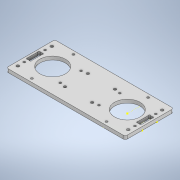
# Autodesk Inventor part: Trunk_waisit_frame_
Saved by Autodesk Inventor 2020.4 (Build 244396000, 396)
## iProperties
Created: 2021-12-30
Part Number: Trunk_waisit_frame_
Material: アルミニウム 2014-T4
Document SubType Name: Modeling
Designer: Masato Kubotera
Density: 2.8 g/cm^3
Appearance: 滑らか - 淡い灰色
Mass: 70.4243 g
Surface Area: 159.281 cm^2
Volume: 25.1515 cm^3
Author: Masato Kubotera
Autodesk Inventor part; units mm, degrees
ref_plane "YZ Plane" through (0, 0, 0) normal (1, 0, 0) x (0, 1, 0)
ref_plane "XZ Plane" through (0, 0, 0) normal (0, 1, 0) x (-1, 0, 0)
ref_plane "XY Plane" through (0, 0, 0) normal (0, 0, 1) x (1, 0, 0)
derived "Outer_support_stand.ipt"
sketch "スケッチ1" plane through (0, 0, 0) normal (0, 0, 1) x (1, 0, 0)
  circle A0 centre (0, 0) radius 18.5 construction
  circle A1 centre (0, 0) radius 20.5 construction
  circle A2 centre (0, 0) radius 20.51 construction
  line L0 (0, 0) -> (0, 24.5) construction
  circle A3 centre (0, 24.5) radius 1.55 construction
  circle A4 centre (0, 24.5) radius 3 construction
  arc A5 (0, 28.5) -> (-3.7147, 25.9835) centre (0, 24.5) ccw construction
  arc A6 (-5.1639, 24.7674) -> (-18.8673, 16.8557) centre (0, 0) ccw construction
  arc A7 (-5.1639, 24.7674) -> (-3.7147, 25.9835) centre (-5.5721, 26.7253) ccw construction
  arc A8 (3.7147, 25.9835) -> (5.1639, 24.7674) centre (5.5721, 26.7253) ccw construction
  arc A9 (3.7147, 25.9835) -> (0, 28.5) centre (0, 24.5) ccw construction
  circle A10 centre (0, 24.5) radius 3.05 construction
  arc A11 (-24.0311, 7.9117) -> (-24.0311, -7.9117) centre (0, 0) ccw construction
  arc A12 (-24.0311, 7.9117) -> (-24.3598, 9.7747) centre (-25.9308, 8.5371) ccw construction
  arc A13 (-24.6817, 14.25) -> (-24.3598, 9.7747) centre (-21.2176, 12.25) ccw construction
  arc A14 (-20.645, 16.2088) -> (-24.6817, 14.25) centre (-21.2176, 12.25) ccw construction
  arc A15 (-20.645, 16.2088) -> (-18.8673, 16.8557) centre (-20.3588, 18.1882) ccw construction
  circle A16 centre (-21.2176, 12.25) radius 3.05 construction
  circle A17 centre (-21.2176, 12.25) radius 1.55 construction
  arc A18 (-18.8673, -16.8557) -> (-5.1639, -24.7674) centre (0, 0) ccw construction
  arc A19 (-18.8673, -16.8557) -> (-20.645, -16.2088) centre (-20.3588, -18.1882) ccw construction
  arc A20 (-24.6817, -14.25) -> (-20.645, -16.2088) centre (-21.2176, -12.25) ccw construction
  arc A21 (-24.3598, -9.7747) -> (-24.6817, -14.25) centre (-21.2176, -12.25) ccw construction
  arc A22 (-24.3598, -9.7747) -> (-24.0311, -7.9117) centre (-25.9308, -8.5371) ccw construction
  circle A23 centre (-21.2176, -12.25) radius 3.05 construction
  circle A24 centre (-21.2176, -12.25) radius 1.55 construction
  arc A25 (5.1639, -24.7674) -> (18.8673, -16.8557) centre (0, 0) ccw construction
  arc A26 (5.1639, -24.7674) -> (3.7147, -25.9835) centre (5.5721, -26.7253) ccw construction
  arc A27 (0, -28.5) -> (3.7147, -25.9835) centre (0, -24.5) ccw construction
  arc A28 (-3.7147, -25.9835) -> (0, -28.5) centre (0, -24.5) ccw construction
  arc A29 (-3.7147, -25.9835) -> (-5.1639, -24.7674) centre (-5.5721, -26.7253) ccw construction
  circle A30 centre (0, -24.5) radius 3.05 construction
  circle A31 centre (0, -24.5) radius 1.55 construction
  arc A32 (24.0311, -7.9117) -> (24.0311, 7.9117) centre (0, 0) ccw construction
  arc A33 (24.0311, -7.9117) -> (24.3598, -9.7747) centre (25.9308, -8.5371) ccw construction
  arc A34 (24.6817, -14.25) -> (24.3598, -9.7747) centre (21.2176, -12.25) ccw construction
  arc A35 (20.645, -16.2088) -> (24.6817, -14.25) centre (21.2176, -12.25) ccw construction
  arc A36 (20.645, -16.2088) -> (18.8673, -16.8557) centre (20.3588, -18.1882) ccw construction
  circle A37 centre (21.2176, -12.25) radius 3.05 construction
  circle A38 centre (21.2176, -12.25) radius 1.55 construction
  arc A39 (18.8673, 16.8557) -> (5.1639, 24.7674) centre (0, 0) ccw construction
  arc A40 (18.8673, 16.8557) -> (20.645, 16.2088) centre (20.3588, 18.1882) ccw construction
  arc A41 (24.6817, 14.25) -> (20.645, 16.2088) centre (21.2176, 12.25) ccw construction
  arc A42 (24.3598, 9.7747) -> (24.6817, 14.25) centre (21.2176, 12.25) ccw construction
  arc A43 (24.3598, 9.7747) -> (24.0311, 7.9117) centre (25.9308, 8.5371) ccw construction
  circle A44 centre (21.2176, 12.25) radius 3.05 construction
  circle A45 centre (21.2176, 12.25) radius 1.55 construction
sketch "スケッチ2" plane through (0, 0, 0) normal (0, 0, 1) x (1, 0, 0)
  line L0 (-114, 28.5) -> (26, 28.5)
  line L1 (26, 28.5) -> (26, -28.5)
  line L2 (26, -28.5) -> (-114, -28.5)
  line L3 (-114, -28.5) -> (-114, 28.5)
  line L4 (-114, 28.5) -> (26, -28.5) construction
  line L5 (26, 28.5) -> (-114, -28.5) construction
  line L6 (-114, 0) -> (26, 0) construction
  line L7 (-44, 28.5) -> (-44, -28.5) construction
  line L8 (18.5, 7.5) -> (23.5, 7.5) construction
  line L9 (23.5, 7.5) -> (23.5, -7.5) construction
  line L10 (23.5, -7.5) -> (18.5, -7.5) construction
  line L11 (18.5, -7.5) -> (18.5, 7.5) construction
  line L12 (18.5, 7.5) -> (23.5, -7.5) construction
  line L13 (23.5, 7.5) -> (18.5, -7.5) construction
  circle A0 centre (21, -20) radius 1.6
  line L14 (18.45, 7.55) -> (23.55, 7.55)
  line L15 (23.55, 7.55) -> (23.55, -7.55)
  line L16 (23.55, -7.55) -> (18.45, -7.55)
  line L17 (18.45, -7.55) -> (18.45, 7.55)
  line L18 (18.45, 7.55) -> (23.55, -7.55) construction
  line L19 (23.55, 7.55) -> (18.45, -7.55) construction
  arc A1 (19.9349, 7.55) -> (18.45, 6.0651) centre (19.1925, 6.8075) ccw
  line L20 (21, 7.5) -> (21, -7.5) construction
  line L21 (18.5, 0) -> (23.5, 0) construction
  arc A2 (23.55, 6.0651) -> (22.0651, 7.55) centre (22.8075, 6.8075) ccw
  arc A3 (18.45, -6.0651) -> (19.9349, -7.55) centre (19.1925, -6.8075) ccw
  arc A4 (22.0651, -7.55) -> (23.55, -6.0651) centre (22.8075, -6.8075) ccw
  circle A5 centre (0, 24.5) radius 1.55 construction
  circle A6 centre (-21.2176, 12.25) radius 1.55 construction
  circle A7 centre (-21.2176, -12.25) radius 1.55 construction
  circle A8 centre (0, -24.5) radius 1.55 construction
  circle A9 centre (21.2176, -12.25) radius 1.55 construction
  circle A10 centre (21.2176, 12.25) radius 1.55 construction
  circle A11 centre (0, 24.5) radius 1.25
  circle A12 centre (-21.2176, 12.25) radius 1.25
  circle A13 centre (-21.2176, -12.25) radius 1.25
  circle A14 centre (0, -24.5) radius 1.25
  circle A15 centre (21.2176, -12.25) radius 1.25
  circle A16 centre (21.2176, 12.25) radius 1.25
  circle A17 centre (21, 20) radius 1.6
  circle A18 centre (-109, -20) radius 1.6
  line L22 (-106.45, 7.55) -> (-111.55, 7.55)
  line L23 (-111.55, 7.55) -> (-111.55, -7.55)
  line L24 (-111.55, -7.55) -> (-106.45, -7.55)
  line L25 (-106.45, -7.55) -> (-106.45, 7.55)
  arc A19 (-106.45, 6.0651) -> (-107.9349, 7.55) centre (-107.1925, 6.8075) ccw
  arc A20 (-110.0651, 7.55) -> (-111.55, 6.0651) centre (-110.8075, 6.8075) ccw
  arc A21 (-107.9349, -7.55) -> (-106.45, -6.0651) centre (-107.1925, -6.8075) ccw
  arc A22 (-111.55, -6.0651) -> (-110.0651, -7.55) centre (-110.8075, -6.8075) ccw
  circle A23 centre (-88, 24.5) radius 1.25
  circle A24 centre (-66.7824, 12.25) radius 1.25
  circle A25 centre (-66.7824, -12.25) radius 1.25
  circle A26 centre (-88, -24.5) radius 1.25
  circle A27 centre (-109.2176, -12.25) radius 1.25
  circle A28 centre (-109.2176, 12.25) radius 1.25
  circle A29 centre (-109, 20) radius 1.6
  circle A30 centre (0, 0) radius 10.5 construction
  line L26 (0, 0) -> (0, 24.5) construction
  line L27 (-31, -16) -> (-31, 16) construction
  line L28 (-31, 16) -> (12, 16) construction
  line L29 (12, 16) -> (12, -16) construction
  line L30 (12, -16) -> (-31, -16) construction
  line L31 (-31, -16) -> (12, 16) construction
  line L32 (-31, 16) -> (12, -16) construction
  line L33 (-31, 0) -> (12, 0) construction
  line L34 (-31, -14.4) -> (-39.5, -14.4) construction
  line L35 (-39.5, -14.4) -> (-39.5, 14.4) construction
  line L36 (-31, 14.4) -> (-39.5, 14.4) construction
  line L37 (-1, -13.5) -> (-1, 13.5) construction
  line L38 (-1, 13.5) -> (-28, 13.5) construction
  line L39 (-28, 13.5) -> (-28, -13.5) construction
  line L40 (-28, -13.5) -> (-1, -13.5) construction
  line L41 (-1, -13.5) -> (-28, 13.5) construction
  line L42 (-1, 13.5) -> (-28, -13.5) construction
  circle A31 centre (-28, -13.5) radius 1.5
  circle A32 centre (-28, 13.5) radius 1.5
  circle A33 centre (-60, -13.5) radius 1.5
  circle A34 centre (-60, 13.5) radius 1.5
  circle A35 centre (0, 0) radius 15
  circle A36 centre (-28, -13.5) radius 2.75 construction
  circle A37 centre (-88, 0) radius 15
  point P0 (-44, 0)
  point P1 (0, 28.5)
  point P2 (0, -28.5)
  point P3 (21, 0)
  point P4 (21, 0)
  point P5 (22.0651, -7.55)
  point P6 (19.9349, -7.55)
  point P7 (18.45, -6.0651)
  point P8 (22.0651, 7.55)
  point P9 (23.55, 6.0651)
  point P10 (23.55, -6.0651)
  point P11 (-110.0651, 7.55)
  point P12 (-106.45, -6.0651)
  point P13 (-107.9349, -7.55)
  point P14 (-110.0651, -7.55)
  point P15 (-111.55, -6.0651)
  point P16 (-111.55, 6.0651)
  point P17 (-9.5, 0)
  point P18 (-14.5, 0)
  dimension "d5" = 5
  dimension "d6" = 15
  dimension "d7" = 3.2
  dimension "d14" = 0.05
  dimension "d15" = 0.05
  dimension "d16" = 1.05
  dimension "d25" = 2.5
  dimension "d26" = 2.5
  dimension "d27" = 2.5
  dimension "d28" = 2.5
  dimension "d29" = 2.5
  dimension "d30" = 2.5
  dimension "d40" = 21
  dimension "d42" = 2.5
  dimension "d43" = 57
  dimension "d44" = 140
  dimension "d45" = 90
  dimension "d46" = 44
  dimension "d47" = 43
  dimension "d48" = 32
  dimension "d49" = 28.8
  dimension "d50" = 8.5
  dimension "d51" = 9.5
  dimension "d52" = 27
  dimension "d53" = 27
  dimension "d54" = 3
  dimension "d55" = 8.5
  dimension "d56" = 180
  dimension "d58" = 40
  dimension "d59" = 30
  dimension "d60" = 3.5
  dimension "d61" = 5.5
  constraints: 84 end point, 40 symmetric about line, 32 centre point, 21 midpoint, 17 point on circle, 12 parallel, 10 point on line, 9 coincident, 7 perpendicular, 20 other
  measures "d5" distance of L9.end L10.end
  measures "d6" distance of L8.end L9.end
  measures "d7" diameter of A0
  measures "d14" distance between parallel lines of L17 L11
  measures "d15" distance between parallel lines of L14 L8
  measures "d16" radius of A1
  measures "d25" diameter of A11
  measures "d26" diameter of A12
  measures "d27" diameter of A13
  measures "d28" diameter of A14
  measures "d29" diameter of A15
  measures "d30" diameter of A16
  measures "d40" diameter of A30
  measures "d42" distance between parallel lines of L9 L1
  measures "d43" distance of L0.end L1.end
  measures "d44" distance of L0.start L0.end
  measures "d45" angle of L0 L26
  measures "d46" distance of A30.centre point (-44, 0)
  measures "d47" distance of L27.end L28.end
  measures "d48" distance of L28.end L29.end
  measures "d49" distance of L34.end L35.end
  measures "d50" distance of L34.start L34.end
  measures "d51" distance of A30.centre point (-9.5, 0)
  measures "d52" distance of L39.end L38.end
  measures "d53" distance of L38.end L37.end
  measures "d54" diameter of A31
  measures "d55" distance from line of point (-9.5, 0) L37
  measures "d56" angle of L26 L27
  measures "d58" distance of A0.centre A17.centre
  measures "d59" diameter of A35
  measures "d60" distance edge to line of A35 L11
  measures "d61" diameter of A36
extrude "押し出し1" add sketch "スケッチ2" along normal blind 4
fillet "フィレット1" radius 2.5 4 edges at (26, 28.5, 2) (26, -28.5, 2) (-114, -28.5, 2) (-114, 28.5, 2)
equation "\"d15\" = d14"
